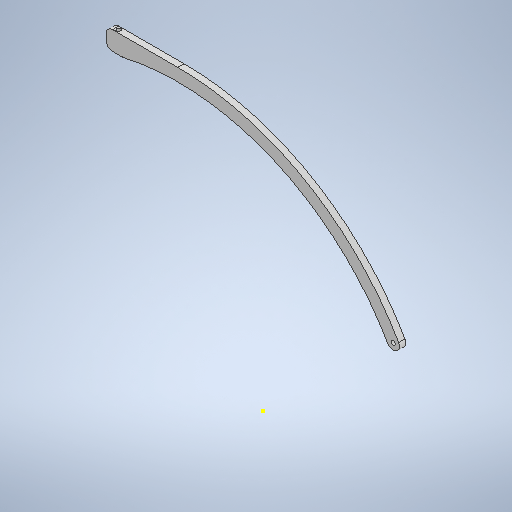
# Autodesk Inventor part: light_ball_space_side
Saved by Autodesk Inventor 2025.1 (Build 291241000, 241)
## iProperties
Created: 2025-05-06
Part Number: light_ball_space_side
Material: 一般
Document SubType Name: Modeling
Designer: yuki0520
Density: 1 g/cm^3
Appearance: 既定
Author: yuki0520
Autodesk Inventor part; units mm, degrees
ref_plane "YZ Plane" through (0, 0, 0) normal (1, 0, 0) x (0, 1, 0)
ref_plane "XZ Plane" through (0, 0, 0) normal (0, 1, 0) x (-1, 0, 0)
ref_plane "XY Plane" through (0, 0, 0) normal (0, 0, 1) x (1, 0, 0)
derived "zzz_light_plate.ipt"
sketch "スケッチ1" plane through (0, 0, 0) normal (0, 0, 1) x (1, 0, 0)
  circle A0 centre (0, 0) radius 120
  line L0 (12.25, 120) -> (-12.25, 120)
  line L1 (-12.25, 120) -> (-12.25, 196)
  line L2 (-12.25, 196) -> (12.25, 196)
  line L3 (12.25, 196) -> (12.25, 120)
  line L4 (12.25, 120) -> (-12.25, 196) construction
  line L5 (-12.25, 120) -> (12.25, 196) construction
  line L6 (-41.25, 158) -> (95.75, 158)
  line L7 (0, -120) -> (0, 120)
  line L8 (56.75, 134) -> (46.75, 134)
  line L9 (46.75, 134) -> (46.75, 182)
  line L10 (46.75, 182) -> (56.75, 182)
  line L11 (56.75, 182) -> (56.75, 134)
  line L12 (56.75, 134) -> (46.75, 182) construction
  line L13 (46.75, 134) -> (56.75, 182) construction
  line L14 (60, 182) -> (50, 182)
  line L15 (53.25, 218) -> (53.25, 138)
  circle A1 centre (400, 0) radius 120
  circle A2 centre (400, 158) radius 38
  line L16 (400, -120) -> (400, 120)
  line L17 (-120, 0) -> (120, 0)
  circle A3 centre (400, 158) radius 17
  circle A4 centre (434, 158) radius 17
  circle A5 centre (434, 158) radius 12
  line L18 (430, 218) -> (415, 218)
  line L19 (415, 218) -> (415, 233)
  line L20 (415, 233) -> (430, 233)
  line L21 (430, 233) -> (430, 218)
  line L22 (385, 138) -> (460, 138)
  line L23 (460, 138) -> (460, 218)
  line L24 (460, 218) -> (385, 218)
  line L25 (385, 218) -> (385, 138)
  line L26 (362, 158) -> (438, 158)
  line L27 (422.5, 233) -> (422.5, 173)
  circle A6 centre (422.5, 173) radius 2
  line L28 (96.25, 146) -> (53.25, 146)
  line L29 (53.25, 146) -> (53.25, 170)
  line L30 (53.25, 170) -> (96.25, 170)
  line L31 (96.25, 170) -> (96.25, 146)
  line L32 (96.25, 146) -> (53.25, 170) construction
  line L33 (53.25, 146) -> (96.25, 170) construction
  line L34 (48.25, 218) -> (48.25, 120)
  circle A7 centre (434, 158) radius 9.5
  circle A8 centre (434, 158) radius 6.55
  circle A9 centre (443.5, 158) radius 1.3
  circle A10 centre (429.25, 166.2272) radius 1.3
  circle A11 centre (429.25, 149.7728) radius 1.3
  line L35 (415, 218) -> (430, 218)
  line L36 (430, 218) -> (430, 203)
  line L37 (430, 203) -> (415, 203)
  line L38 (415, 203) -> (415, 218)
  line L39 (125, 218) -> (-125, 218)
  line L40 (-125, 218) -> (-125, 203)
  line L41 (-125, 203) -> (125, 203)
  line L42 (125, 203) -> (125, 218)
  circle A12 centre (400, 158) radius 9
  circle A13 centre (422.5, 203) radius 1.6
  circle A14 centre (434, 158) radius 7.5
  line L43 (-33.25, 218) -> (-33.25, 138)
  line L44 (20.25, 218) -> (20.25, 138)
  line L45 (15.25, 138) -> (15.25, 218)
  line L46 (-28.25, 218) -> (-28.25, 138)
  circle A15 centre (428.45, 203) radius 1.55
  circle A16 centre (416.55, 203) radius 1.55
  line L47 (12.25, -196) -> (12.25, -120)
  line L48 (12.25, -120) -> (-12.25, -196) construction
  line L49 (-12.25, -120) -> (-12.25, -196)
  line L50 (12.25, -120) -> (-12.25, -120)
  line L51 (-12.25, -120) -> (12.25, -196) construction
  line L52 (-12.25, -196) -> (12.25, -196)
  line L53 (15.25, -138) -> (15.25, -218)
  line L54 (-41.25, -158) -> (95.75, -158)
  line L55 (-125, -203) -> (125, -203)
  line L56 (125, -218) -> (-125, -218)
  line L57 (48.25, -218) -> (48.25, -120)
  line L58 (125, -203) -> (125, -218)
  line L59 (53.25, -218) -> (53.25, -138)
  line L60 (20.25, -218) -> (20.25, -138)
  line L61 (53.25, -146) -> (53.25, -170)
  line L62 (96.25, -146) -> (53.25, -146)
  line L63 (96.25, -146) -> (53.25, -170) construction
  line L64 (96.25, -170) -> (96.25, -146)
  line L65 (53.25, -146) -> (96.25, -170) construction
  line L66 (-33.25, -218) -> (-33.25, -138)
  line L67 (-125, -218) -> (-125, -203)
  line L68 (-28.25, -218) -> (-28.25, -138)
  line L69 (46.75, -182) -> (56.75, -182)
  line L70 (60, -182) -> (50, -182)
  line L71 (53.25, -170) -> (96.25, -170)
  line L72 (46.75, -134) -> (56.75, -182) construction
  line L73 (56.75, -134) -> (46.75, -134)
  line L74 (56.75, -182) -> (56.75, -134)
  line L75 (46.75, -134) -> (46.75, -182)
  line L76 (56.75, -134) -> (46.75, -182) construction
  circle A17 centre (422.5, 204.5) radius 1.6
  circle A18 centre (434, 158) radius 23
  circle A19 centre (455.7428, 150.5) radius 2.05
  circle A20 centre (429.6238, 180.5798) radius 2.05
  circle A21 centre (416.6334, 142.9202) radius 2.05
  circle A22 centre (416.6334, 142.9202) radius 3
  line L77 (-125, 203) -> (-125, -203)
  point P0 (0, 158)
  point P1 (51.75, 158)
  point P2 (74.75, 158)
  point P3 (0, -158)
  point P4 (51.75, -158)
  point P5 (74.75, -158)
sketch "スケッチ2" plane through (0, 0, 0) normal (0, 0, 1) x (1, 0, 0)
  line L0 (12.25, 120) -> (-12.25, 120) projected
  line L1 (56.75, 134) -> (46.75, 134) projected
  line L2 (-41.25, 158) -> (95.75, 158) projected
  line L3 (46.75, 134) -> (46.75, 182) projected
  line L4 (60, 182) -> (50, 182) projected
  line L5 (56.75, 134) -> (46.75, 182) construction
  line L6 (46.75, 182) -> (56.75, 182) projected
  line L7 (56.75, 182) -> (56.75, 134) projected
  line L8 (46.75, 134) -> (56.75, 182) construction
  line L9 (12.25, 196) -> (12.25, 120) projected
  line L10 (-12.25, 120) -> (12.25, 196) construction
  line L11 (-12.25, 120) -> (-12.25, 196) projected
  line L12 (12.25, 120) -> (-12.25, 196) construction
  line L13 (-12.25, 196) -> (12.25, 196) projected
  circle A0 centre (0, 0) radius 120 projected
  line L14 (-120, 0) -> (120, 0) projected
  line L15 (-125, 203) -> (-125, -203) projected
  line L16 (0, -120) -> (0, 120) projected
  circle A1 centre (400, 0) radius 120 projected
  line L17 (400, -120) -> (400, 120) projected
  circle A2 centre (434, 158) radius 6.55 projected
  circle A3 centre (434, 158) radius 7.5 projected
  circle A4 centre (434, 158) radius 9.5 projected
  line L18 (96.25, 146) -> (53.25, 146) projected
  line L19 (53.25, 146) -> (53.25, 170) projected
  line L20 (53.25, 170) -> (96.25, 170) projected
  line L21 (96.25, 170) -> (96.25, 146) projected
  line L22 (53.25, 146) -> (96.25, 170) construction
  line L23 (96.25, 146) -> (53.25, 170) construction
  line L24 (430, 218) -> (415, 218) projected
  line L25 (415, 218) -> (415, 233) projected
  line L26 (415, 233) -> (430, 233) projected
  line L27 (430, 233) -> (430, 218) projected
  line L28 (422.5, 233) -> (422.5, 173) projected
  line L29 (430, 203) -> (415, 203) projected
  circle A5 centre (428.45, 203) radius 1.55 projected
  circle A6 centre (416.55, 203) radius 1.55 projected
  circle A7 centre (422.5, 203) radius 1.6 projected
  circle A8 centre (422.5, 204.5) radius 1.6 projected
  line L30 (415, 218) -> (430, 218) projected
  line L31 (415, 203) -> (415, 218) projected
  line L32 (430, 218) -> (430, 203) projected
  line L33 (-125, 203) -> (125, 203) projected
  line L34 (125, 218) -> (-125, 218) projected
  line L35 (-125, 218) -> (-125, 203) projected
  line L36 (125, 203) -> (125, 218) projected
  line L37 (53.25, 218) -> (53.25, 138) projected
  line L38 (48.25, 218) -> (48.25, 120) projected
  line L39 (-33.25, 218) -> (-33.25, 138) projected
  line L40 (-28.25, 218) -> (-28.25, 138) projected
  line L41 (15.25, 138) -> (15.25, 218) projected
  line L42 (20.25, 218) -> (20.25, 138) projected
  line L43 (15.25, -138) -> (15.25, -218) projected
  line L44 (20.25, -218) -> (20.25, -138) projected
  line L45 (53.25, -218) -> (53.25, -138) projected
  line L46 (48.25, -218) -> (48.25, -120) projected
  line L47 (46.75, -182) -> (56.75, -182) projected
  line L48 (60, -182) -> (50, -182) projected
  line L49 (46.75, -134) -> (46.75, -182) projected
  line L50 (46.75, -134) -> (56.75, -182) construction
  line L51 (56.75, -182) -> (56.75, -134) projected
  line L52 (56.75, -134) -> (46.75, -182) construction
  line L53 (56.75, -134) -> (46.75, -134) projected
  line L54 (53.25, -146) -> (53.25, -170) projected
  line L55 (96.25, -146) -> (53.25, -146) projected
  line L56 (96.25, -170) -> (96.25, -146) projected
  line L57 (96.25, -146) -> (53.25, -170) construction
  line L58 (53.25, -146) -> (96.25, -170) construction
  line L59 (125, -203) -> (125, -218) projected
  line L60 (53.25, -170) -> (96.25, -170) projected
  line L61 (12.25, -120) -> (-12.25, -120) projected
  line L62 (-41.25, -158) -> (95.75, -158) projected
  line L63 (12.25, -196) -> (12.25, -120) projected
  line L64 (-12.25, -120) -> (12.25, -196) construction
  line L65 (-12.25, -120) -> (-12.25, -196) projected
  line L66 (12.25, -120) -> (-12.25, -196) construction
  line L67 (-12.25, -196) -> (12.25, -196) projected
  line L68 (-125, -203) -> (125, -203) projected
  line L69 (125, -218) -> (-125, -218) projected
  line L70 (-33.25, -218) -> (-33.25, -138) projected
  line L71 (-125, -218) -> (-125, -203) projected
  line L72 (-28.25, -218) -> (-28.25, -138) projected
  circle A9 centre (400, 158) radius 38 projected
  circle A10 centre (400, 158) radius 17 projected
  circle A11 centre (434, 158) radius 17 projected
  circle A12 centre (434, 158) radius 12 projected
  circle A13 centre (429.25, 166.2272) radius 1.3 projected
  circle A14 centre (429.25, 149.7728) radius 1.3 projected
  circle A15 centre (443.5, 158) radius 1.3 projected
  circle A16 centre (422.5, 173) radius 2 projected
  circle A17 centre (455.7428, 150.5) radius 2.05 projected
  circle A18 centre (429.6238, 180.5798) radius 2.05 projected
  circle A19 centre (416.6334, 142.9202) radius 2.05 projected
  circle A20 centre (416.6334, 142.9202) radius 3 projected
  line L73 (362, 158) -> (438, 158) projected
  circle A21 centre (400, 158) radius 9 projected
  line L74 (460, 138) -> (460, 218) projected
  line L75 (385, 218) -> (385, 138) projected
  line L76 (460, 218) -> (385, 218) projected
  line L77 (385, 138) -> (460, 138) projected
  circle A22 centre (434, 158) radius 23 projected
  arc A23 (-125, -179.1508) -> (-125, 179.1508) centre (-68, 0) ccw
  line L78 (-125, 203) -> (125, 203)
  line L79 (125, 203) -> (125, 188)
  line L80 (125, 188) -> (-125, 188)
  line L81 (-125, 188) -> (-125, 203)
  arc A24 (-136.776, -190.9944) -> (-136.776, 190.9944) centre (-68, 0) ccw
  arc A25 (-133.388, -181.5858) -> (-133.388, 181.5858) centre (-68, 0) ccw
  line L82 (-129.5521, 193) -> (-33.25, 193)
  line L83 (0, 0) -> (110, 97.5961)
  line L84 (110, 218) -> (110, 188)
  point P0 (0, 158)
  point P1 (51.75, 158)
  point P2 (74.75, 158)
  point P3 (51.75, -158)
  point P4 (74.75, -158)
  point P5 (0, -158)
  point P6 (42.8377, 158)
  point P7 (48.25, 158)
  point P8 (48.25, 154.0615)
  point P9 (58.226, -146)
  point P10 (73.0425, -146)
  point P11 (-68, 203)
  point P12 (-125, 188)
  point P13 (-111.6463, 188)
  point P14 (102.3174, 90.7798)
  dimension "d1" = 15
  dimension "d2" = 15
  dimension "d3" = 5
  dimension "d24" = 15
  constraints: 14 end point, 7 point on circle, 6 point on line, 3 centre point, 3 perpendicular, 3 tangent, 2 horizontal alignment, 2 parallel, 1 collinear, 1 horizontal, 3 other
  measures "d1" distance of L78.end L79.end
  measures "d2" radial gap between concentric circles of A23 A24
  measures "d3" radial gap between concentric circles of A23 A25
  measures "d24" distance between parallel lines of L36 L84
extrude "押し出し1" add sketch "スケッチ2" along normal blind 5 contours A25 L11 L80 A24 L9 | L9 A24 L41 A25 | A25 L18 A24 L83 | A25 L80 L11 | L41 A24 L42 A25 | A25 L7 L2 A24 L18 | L80 A25 L40 A24 L11 | L11 A24 L80 | A25 L42 A24 L3 L2 | L2 L3 A25 | A25 L19 L2 L7 | A25 L39 A24 L40 | L3 A24 L38 L2 | L2 L38 A25 L3 | L7 A24 L2 | L2 L19 A24 L7 | A25 L38 L2 L19 | A25 L82 L39 | L80 L15 L82 A25 | L38 A24 L19 L2 | L82 L15 A24 L39 | A24 L15 L33
sketch "スケッチ3" plane through (-125, 203, 0) normal (0, 1, 0) x (1, 0, 0)
  line L0 (57, 0) -> (0, 0) projected
  line L1 (0, 0) -> (0, -5) projected
  line L2 (57, -5) -> (0, -5) projected
  line L3 (57, 0) -> (57, -5) projected
  line L4 (0, -2.5) -> (57, -2.5)
  point P0 (125, 0)
  point P1 (7.5, -2.5)
  dimension "d6" = 7.5
  constraints: 2 end point, 2 midpoint, 1 point on line
  measures "d6" horizontal distance of L0.end point (7.5, -2.5)
hole "穴1" at (-117.5, 203, 2.5) direction (0, -1, 0) diameter 3.2 end through all
sketch "スケッチ4" plane through (0, 0, 5) normal (0, 0, 1) x (1, 0, 0)
  circle A0 centre (-117.5, 204.5) radius 1.6
  line L0 (-68, 203) -> (-125, 203) projected
  line L1 (-118.0568, 203) -> (-116.9432, 203)
  line L2 (-117.5, 203) -> (-117.5, 186.5442)
  arc A1 (102.3174, 90.7798) -> (-111.6463, 188) centre (-68, 0) ccw projected
  line L3 (-125, 203) -> (-125, 188) projected
  point P0 (0, 0)
  point P1 (-115.9, 203)
  point P2 (42.8377, 158)
  dimension "d14" = 3.2
  dimension "d15" = 1.5
  dimension "d18" = 7.5
  constraints: 4 end point, 4 point on line, 3 point on circle, 1 centre point, 1 vertical
  measures "d14" diameter of A0
  measures "d15" distance from line of L0 A0.centre
  measures "d18" distance between parallel lines of L3 L2
extrude "押し出し2" cut sketch "スケッチ4" against normal blind 5 contours L0 L2 A0 | A0 L2 L0
fillet "フィレット1" radius 5 5 edges at (-125, 203, 2.5) (-125, 188, 2.5) (-111.6463, 188, 2.5) (110, 97.5961, 2.5) (102.3174, 90.7798, 2.5)
sketch "スケッチ5" plane through (0, 0, 5) normal (0, 0, 1) x (1, 0, 0)
  arc A0 (99.3326, 96.1706) -> (108.0027, 101.1536) centre (103.6677, 98.6621) ccw projected
  arc A1 (108.0027, 101.1536) -> (-68, 203) centre (-68, 0) ccw projected
  line L0 (-68, 203) -> (-116.9432, 203) projected
  arc A2 (-118.0568, 203) -> (-116.9432, 203) centre (-117.5, 204.5) ccw projected
  line L1 (-118.0568, 203) -> (-120, 203) projected
  arc A3 (-120, 203) -> (-125, 198) centre (-120, 198) ccw projected
  line L2 (-125, 198) -> (-125, 193) projected
  arc A4 (-112.2154, 188) -> (-111.0988, 188.1263) centre (-112.2154, 193) ccw projected
  arc A5 (99.3326, 96.1706) -> (-111.0988, 188.1263) centre (-68, 0) ccw projected
  circle A6 centre (103.6677, 98.6621) radius 1.6
  line L3 (-120, 0) -> (120, 0) projected
  arc A7 (99.3326, 96.1706) -> (-111.0988, 188.1263) centre (-68, 0) ccw
  arc A8 (84.8931, 125.8082) -> (-125, 189.618) centre (-68, 0) ccw
  line L4 (96.25, 146) -> (53.25, 146) projected
  line L5 (99.3326, 96.1706) -> (108.0027, 101.1536)
  arc A9 (-125, 193) -> (-120, 188) centre (-120, 193) ccw projected
  line L6 (-120, 188) -> (-112.2154, 188) projected
  point P0 (0, 0)
  dimension "d20" = 3.2
  dimension "d21" = 5
  constraints: 5 point on circle, 3 centre point, 2 end point, 1 midpoint
  measures "d20" diameter of A6
  measures "d21" radial gap between concentric circles of A7 A8
extrude "押し出し3" cut sketch "スケッチ5" against normal blind 5 contours L5 A6 | A6 L5
sketch "スケッチ7" plane through (0, 0, 5) normal (0, 0, 1) x (1, 0, 0)
  point P0 (0, 0)
